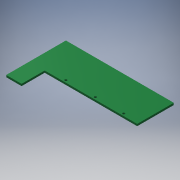
# Autodesk Inventor part: IR_PCB_Inventor
Saved by Autodesk Inventor 2018 (Build 220112000, 112)
## iProperties
Created: 2018-02-04
Part Number: IR_PCB_Inventor
Material: Generic
Document SubType Name: Modeling
Designer: Mandus
Density: 1 g/cm^3
Appearance: Default
Author: Mandus
Autodesk Inventor part; units mm, degrees
ref_plane "YZ Plane" through (0, 0, 0) normal (1, 0, 0) x (0, 1, 0)
ref_plane "XZ Plane" through (0, 0, 0) normal (0, 1, 0) x (-1, 0, 0)
ref_plane "XY Plane" through (0, 0, 0) normal (0, 0, 1) x (1, 0, 0)
sketch "Sketch1" plane through (0, 0, 0) normal (0, 0, 1) x (1, 0, 0)
  circle A0 centre (119.5, -44.5) radius 1.5
  circle A1 centre (82.7, -44.5) radius 1.5
  circle A2 centre (44.5, -44.5) radius 1.5
  line L0 (0, 0) -> (140, 0)
  line L1 (140, 0) -> (140, -47.5)
  line L2 (140, -47.5) -> (0, -47.5)
  line L3 (0, -47.5) -> (0, 0)
  line L4 (0, -47.5) -> (20, -47.5)
  line L5 (20, -47.5) -> (20, -77.5)
  line L6 (20, -77.5) -> (0, -77.5)
  line L7 (0, -77.5) -> (0, -47.5)
  dimension "d8" = 3
  dimension "d10" = 36.8
  dimension "d11" = 75
  dimension "d15" = 140
  dimension "d16" = 47.5
  dimension "d17" = 20
  dimension "d18" = 30
  constraints: 16 end point, 4 parallel, 3 centre point, 2 equal radius, 2 horizontal, 2 horizontal alignment, 2 perpendicular
  measures "d8" diameter of A0
  measures "d10" distance of A1.centre A0.centre
  measures "d11" distance of A2.centre A0.centre
  measures "d15" distance of L1.end L2.end
  measures "d16" distance of L0.end L1.end
  measures "d17" distance of L5.end L6.end
  measures "d18" distance of L4.end L5.end
extrude "Extrusion1" add sketch "Sketch1" along normal blind 2.5
body "Solid1"
